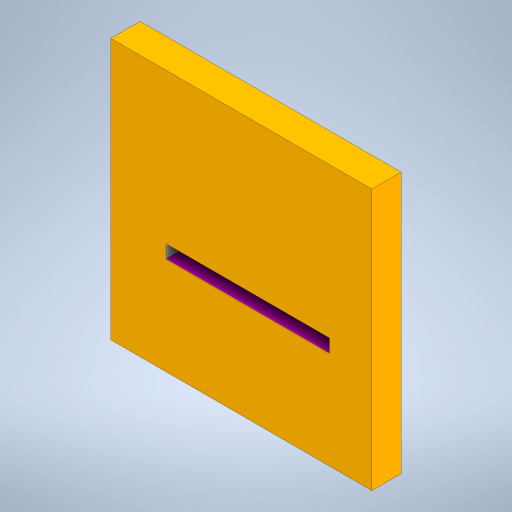
# Autodesk Inventor part: basebottomds
Saved by Autodesk Inventor 2024 (Build 280153000, 153)
## iProperties
Created: 2023-06-04
Part Number: basebottomds
Material: Generic
Document SubType Name: Modeling
Designer: hithi
Density: 1 g/cm^3
Appearance: Default
Author: hithi
Autodesk Inventor part; units mm, degrees
ref_plane "YZ Plane" through (0, 0, 0) normal (1, 0, 0) x (0, 1, 0)
ref_plane "XZ Plane" through (0, 0, 0) normal (0, 1, 0) x (-1, 0, 0)
ref_plane "XY Plane" through (0, 0, 0) normal (0, 0, 1) x (1, 0, 0)
sketch "Sketch1" plane through (0, 0, 0) normal (0, 0, 1) x (1, 0, 0)
  line L0 (0, 0) -> (400, 0)
  line L1 (400, 0) -> (400, 400)
  line L2 (400, 400) -> (0, 400)
  line L3 (0, 400) -> (0, 0)
  line L4 (135, 150) -> (335, 150)
  line L5 (335, 150) -> (335, 170)
  line L6 (335, 170) -> (135, 170)
  line L7 (135, 170) -> (135, 150)
  dimension "d0" = 400
  dimension "d1" = 400
  dimension "d2" = 200
  dimension "d3" = 20
  constraints: 16 end point, 4 parallel, 2 horizontal, 2 perpendicular
  measures "d0" distance of L2.end L1.end
  measures "d1" distance of L1.end L0.end
  measures "d2" distance of L6.end L5.end
  measures "d3" distance of L5.end L4.end
extrude "Extrusion1" add sketch "Sketch1" along normal blind 40
sketch "Sketch2" plane through (0, 0, 0) normal (0, 0, -1) x (-1, 0, 0)
  line L0 (-400, 0) -> (-400, 400) projected
  line L1 (0, 400) -> (-400, 400)
  line L2 (-400, 400) -> (-400, 0)
  line L3 (-400, 0) -> (0, 0)
  line L4 (0, 0) -> (0, 400)
  constraints: 8 end point, 2 parallel, 1 horizontal, 1 perpendicular
extrude "Extrusion2" add sketch "Sketch2" along normal blind 5
sketch "Sketch3" plane through (0, 0, 40) normal (0, 0, 1) x (1, 0, 0)
  line L0 (335, 150) -> (135, 150) projected
  line L1 (135, 150) -> (85, 150)
  line L2 (85, 150) -> (85, 170)
  line L3 (85, 170) -> (135, 170)
  line L4 (135, 170) -> (135, 150)
  point P0 (0, 0)
  dimension "d8" = 50
  dimension "d9" = 20
  constraints: 8 end point, 2 parallel, 1 horizontal, 1 perpendicular
  measures "d8" distance of L2.end L3.end
  measures "d9" distance of L1.end L2.end
extrude "Extrusion3" cut sketch "Sketch3" against normal blind 40
body "Solid1"
